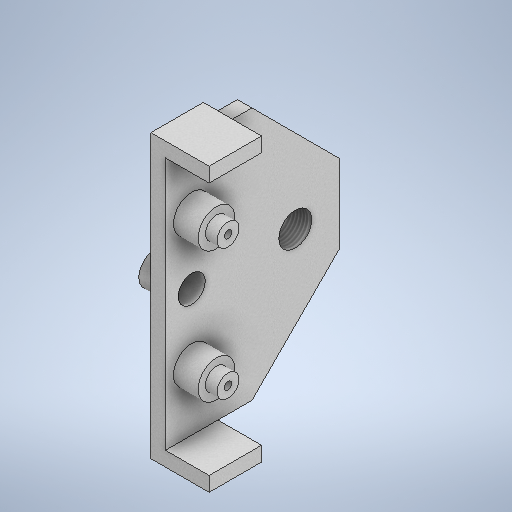
# Autodesk Inventor part: Führungsplatte_rechts
Saved by Autodesk Inventor 2025.2 (Build 292293000, 293)
## iProperties
Created: 2025-02-03
Part Number: Führungsplatte_rechts
Material: Generisch
Document SubType Name: Modeling
Designer: unter
Density: 1 g/cm^3
Appearance: Vorgabe
Author: unter
Autodesk Inventor part; units mm, degrees
ref_plane "YZ Plane" through (0, 0, 0) normal (1, 0, 0) x (0, 1, 0)
ref_plane "XZ Plane" through (0, 0, 0) normal (0, 1, 0) x (-1, 0, 0)
ref_plane "XY Plane" through (0, 0, 0) normal (0, 0, 1) x (1, 0, 0)
derived "Skelett_Laufkatze.ipt"
sketch "Fuehrungsplatte_seite_Kettenzug" plane through (-131, 0, 0) normal (1, 0, 0) x (0, 1, 0)
  line L0 (174, 98.4) -> (-174, 98.4)
  line L1 (-174, -20.4) -> (-54, -140.4)
  line L2 (-54, -140.4) -> (54, -140.4)
  line L3 (54, -140.4) -> (174, -20.4)
  line L4 (0, 8.4) -> (0, 0) construction
  line L5 (1500, 8.4) -> (-1500, 8.4) construction
  circle A0 centre (90, 62.4) radius 54 construction
  circle A1 centre (-90, 62.4) radius 54 construction
  circle A2 centre (0, 62.4) radius 36 construction
  circle A3 centre (90, 62.4) radius 25
  circle A4 centre (-90, 62.4) radius 25
  circle A5 centre (90, 62.4) radius 15
  circle A6 centre (-90, 62.4) radius 15
  circle A7 centre (0, -80) radius 33.75
  circle A8 centre (0, -80) radius 22.5
  line L6 (174, 98.4) -> (194, 98.4)
  line L7 (194, 98.4) -> (194, 26.4)
  line L8 (194, 26.4) -> (174, 26.4)
  line L9 (-174, 98.4) -> (-194, 98.4)
  line L10 (-194, 98.4) -> (-194, 26.4)
  line L11 (-194, 26.4) -> (-174, 26.4)
  circle A9 centre (0, 62.4) radius 22.5
  circle A10 centre (0, 62.4) radius 18.5
  line L12 (174, 26.4) -> (174, -20.4)
  line L13 (-174, 26.4) -> (-174, -20.4)
  point P0 (0, 0)
  point P1 (0, 0)
  point P2 (0, 98.4)
  point P3 (0, -140.4)
sketch "Fuehrungsplatte_Laufradaufhängung_Kettenzug" plane through (-131, 0, 62.4) normal (0, 0, -1) x (-1, 0, 0)
  line L0 (0, -65) -> (0, -115) construction
  line L1 (0, -75) -> (0, -105) construction
  line L2 (0, 22.5) -> (0, -22.5) construction
  line L3 (0, 18.5) -> (0, -18.5) construction
  line L4 (0, 115) -> (0, 65) construction
  line L5 (0, 105) -> (0, 75) construction
  line L6 (0, 174) -> (0, -174)
  line L7 (0, -174) -> (0, -194)
  line L8 (0, 174) -> (0, 194)
  line L9 (0, 194) -> (20, 194)
  line L10 (20, -194) -> (0, -194)
  line L11 (0, -65) -> (-34, -65)
  line L12 (0, -115) -> (-34, -115)
  line L13 (-34, -105) -> (-50, -105)
  line L14 (-34, -75) -> (-50, -75)
  line L15 (-34, -115) -> (-34, -65)
  line L16 (-50, -75) -> (-50, -105)
  line L17 (0, 115) -> (-34, 115)
  line L18 (-34, 115) -> (-34, 65)
  line L19 (-34, 65) -> (0, 65)
  line L20 (-34, 75) -> (-50, 75)
  line L21 (-50, 75) -> (-50, 105)
  line L22 (-50, 105) -> (-34, 105)
  line L23 (0, 22.5) -> (50, 22.5)
  line L24 (0, 18.5) -> (50, 18.5)
  line L25 (0, -18.5) -> (50, -18.5)
  line L26 (0, -22.5) -> (50, -22.5)
  line L27 (50, -22.5) -> (50, 22.5)
  line L28 (20, 194) -> (20, 22.5)
  line L29 (20, -22.5) -> (20, -194)
  line L30 (0, 194) -> (-60, 194)
  line L31 (-60, 194) -> (-60, 174)
  line L32 (-60, 174) -> (0, 174)
  line L33 (0, 174) -> (0, 194)
  line L34 (0, -174) -> (-60, -174)
  line L35 (-60, -174) -> (-60, -194)
  line L36 (-60, -194) -> (0, -194)
  line L37 (0, -194) -> (0, -174)
  point P0 (-131, 0)
sketch "Fuehrungsplatte_Schraubbolzen_Kettenzug" plane through (-131, 0, -80) normal (0, 0, -1) x (-1, 0, 0)
  line L0 (0, 33.75) -> (0, -33.75)
  line L1 (0, 22.5) -> (0, -22.5)
  line L2 (0, 33.75) -> (50, 33.75)
  line L3 (50, 33.75) -> (50, -33.75)
  line L4 (50, -33.75) -> (0, -33.75)
  line L5 (0, 22.5) -> (50, 22.5)
  line L6 (0, -22.5) -> (50, -22.5)
  point P0 (-131, 0)
extrude "Grundplatte" add sketch "Fuehrungsplatte_seite_Kettenzug" against normal up to surface (20 mm away) contours L6 L7 L8 L12 L3 L2 L1 L13 L11 L10 L9 L0
extrude "Wellenöffnung_für_Kettenzug" add sketch "Fuehrungsplatte_seite_Kettenzug" against normal up to surface (50 mm away) from surface at 0 contours A9
extrude "Laufradaufhängung_1" add sketch "Fuehrungsplatte_seite_Kettenzug" along normal up to surface (54 mm away) from surface at -20 contours A3 | A4
extrude "Laufradaufhängung_2" add sketch "Fuehrungsplatte_seite_Kettenzug" along normal up to surface (70 mm away) from surface at -20 contours A5 | A6
extrude "Schutzwände" add sketch "Fuehrungsplatte_Laufradaufhängung_Kettenzug" along normal up to surface (72 mm away) from surface at -36 contours L32 L31 L30 L8 | L7 L36 L35 L34
extrude "Schraubbolzenöffnung" add sketch "Fuehrungsplatte_seite_Kettenzug" against normal up to surface (50 mm away) from surface at 0 contours A7
thread "Schraubbolzengewinde" size "M45x4.5" class "6H" standard "ANSI Metric M Profile" full length
ref_plane "Arbeitsebene1" through (-81, -90, 62.4) normal (1, 0, 0) x (0, 0, -1)
sketch "Skizze4" plane through (-81, -90, 62.4) normal (1, 0, 0) x (0, 0, -1)
  circle A0 centre (0, 0) radius 15 projected
  circle A1 centre (0, 180) radius 15 projected
  point P0 (62.4, 90)
  dimension "d6" = 0
  constraints: 2 coincident
hole "Bohrung1" at (-81, -90, 62.4) at (-81, 90, 62.4) direction (-1, 0, 0) diameter 10.106 depth 32.3 tip angle 118 thread size "M12x1.75" class "6H" standard "ISO Metric profile"
